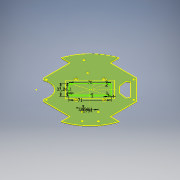
# Autodesk Inventor part: Board1.2
Saved by Autodesk Inventor 2020 (Build 240168000, 168)
## iProperties
Created: 2024-09-20
Part Number: Board1.2
Material: Типовые
Document SubType Name: Modeling
Designer: Ivan
Density: 1 g/cm^3
Appearance: Оливково-зеленый
Author: Ivan
Autodesk Inventor part; units mm, degrees
ref_plane "YZ Plane" through (0, 0, 0) normal (1, 0, 0) x (0, 1, 0)
ref_plane "XZ Plane" through (0, 0, 0) normal (0, 1, 0) x (-1, 0, 0)
ref_plane "XY Plane" through (0, 0, 0) normal (0, 0, 1) x (1, 0, 0)
sketch "Эскиз1" plane through (0, 0, 0) normal (0, 1, 0) x (-1, 0, 0)
  line L0 (-42.0023, -27.4404) -> (-27.4404, -42.0023)
  line L1 (-27.4404, -42.0023) -> (-25.1696, -59.5377)
  line L2 (-25.1696, -59.5377) -> (-32.6924, -63.2376)
  line L3 (-32.6924, -63.2376) -> (-63.2376, -32.6924)
  line L4 (-63.2376, -32.6924) -> (-59.5377, -25.1696)
  line L5 (-59.5377, -25.1696) -> (-42.0023, -27.4404)
  circle A0 centre (-72.43, 16) radius 3.3 construction
  circle A1 centre (44.87, -82.9015) radius 3.3 construction
  circle A2 centre (42.22, 16) radius 3.3
  circle A3 centre (-44.87, 82.9015) radius 3.3 construction
  circle A4 centre (-42.22, 16) radius 3.3 construction
  circle A5 centre (-82.9015, 44.87) radius 3.3 construction
  circle A6 centre (-16, 42.22) radius 3.3 construction
  circle A7 centre (72.43, -16) radius 3.3 construction
  circle A8 centre (16, -72.43) radius 3.3 construction
  circle A9 centre (-16, -72.43) radius 3.3 construction
  circle A10 centre (-42.22, -16) radius 3.3 construction
  circle A11 centre (16, -42.22) radius 3.3 construction
  circle A12 centre (16, 42.22) radius 3.3
  circle A13 centre (16, 72.43) radius 3.3 construction
  circle A14 centre (42.22, -16) radius 3.3 construction
  circle A15 centre (72.43, 16) radius 3.3 construction
  circle A16 centre (-16, 72.43) radius 3.3 construction
  circle A17 centre (82.9015, -44.87) radius 3.3 construction
  circle A18 centre (-16, -42.22) radius 3.3 construction
  circle A19 centre (-72.43, -16) radius 3.3 construction
  line L6 (31, 78.7724) -> (-31, 78.7724)
  line L7 (-31, 78.7724) -> (-31, 99.2724)
  arc A20 (-31, 99.2724) -> (-99.2724, 31) centre (0, 0) ccw
  line L8 (-99.2724, 31) -> (-78.7724, 31)
  line L9 (-78.7724, 31) -> (-78.7724, -31)
  line L10 (-78.7724, -31) -> (-99.2724, -31)
  arc A21 (-99.2724, -31) -> (-98.0863, -34.57) centre (0, 0) ccw
  arc A22 (-34.57, -98.0863) -> (-98.0863, -34.57) centre (-109.0212, -109.0212) ccw
  arc A23 (-34.57, -98.0863) -> (-31, -99.2724) centre (0, 0) ccw
  line L11 (-31, -99.2724) -> (-31, -78.7724)
  line L12 (-31, -78.7724) -> (31, -78.7724)
  line L13 (31, -78.7724) -> (31, -99.2724)
  arc A24 (31, -99.2724) -> (99.2724, -31) centre (0, 0) ccw
  line L14 (99.2724, -31) -> (78.7724, -31)
  line L15 (78.7724, -31) -> (78.7724, 31)
  line L16 (78.7724, 31) -> (99.2724, 31)
  arc A25 (99.2724, 31) -> (98.0863, 34.57) centre (0, 0) ccw
  arc A26 (34.57, 98.0863) -> (98.0863, 34.57) centre (109.0212, 109.0212) ccw
  arc A27 (34.57, 98.0863) -> (31, 99.2724) centre (0, 0) ccw
  line L17 (31, 99.2724) -> (31, 78.7724)
  circle A28 centre (31, 72.43) radius 1.5
  circle A29 centre (72.43, 31) radius 1.5
  circle A30 centre (0, 0) radius 20
  circle A31 centre (-72.43, -31) radius 1.5
  circle A32 centre (-31, -72.43) radius 1.5
  line L18 (-55.8614, 32.5269) -> (-79.196, 55.8614)
  line L19 (-79.196, 55.8614) -> (-55.8614, 79.196)
  line L20 (-55.8614, 79.196) -> (-32.5269, 55.8614)
  line L21 (-32.5269, 55.8614) -> (-55.8614, 32.5269)
  line L22 (48.3138, -22.4528) -> (80.4592, -54.5982)
  line L23 (80.4592, -54.5982) -> (54.5982, -80.4592)
  line L24 (54.5982, -80.4592) -> (22.4528, -48.3138)
  line L25 (22.4528, -48.3138) -> (48.3138, -22.4528)
  line L26 (31, 78.7724) -> (78.7724, 31)
  circle A33 centre (31, 72.43) radius 3.5 construction
  circle A34 centre (72.43, 31) radius 1.5 construction
  circle A35 centre (72.43, 31) radius 3.5 construction
  arc A36 (35.3732, 74.3992) -> (74.3992, 35.3732) centre (63.1933, 63.1933) ccw
  line L27 (-47.7297, -10.253) -> (10.253, 47.7297)
  line L28 (10.253, 47.7297) -> (47.7297, 10.253)
  line L29 (47.7297, 10.253) -> (-10.253, -47.7297)
  line L30 (-10.253, -47.7297) -> (-47.7297, -10.253)
  line L31 (-32.5269, 55.8614) -> (-55.8614, 32.5269) construction
  line L32 (-47.7297, -10.253) -> (47.7297, 10.253) construction
  line L33 (-78.7724, -31) -> (-31, -78.7724)
  dimension "d0" = 7
  dimension "d1" = 7
  dimension "d2" = 82
  dimension "d3" = 53
  constraints: 68 end point, 37 centre point, 18 point on circle, 4 coincident, 3 parallel, 2 point on line, 2 tangent, 1 midpoint, 1 perpendicular
  measures "d0" diameter of A33
  measures "d1" diameter of A35
  measures "d2" distance of L28.end L29.end
  measures "d3" distance of L27.end L28.end
extrude "Выдавливание1" add sketch "Эскиз1" along normal blind 1.6 contours A2 L28 | L28 A12 | L26 A36 L15 L14 A24 L13 L12 L33 L9 L8 A20 L7 L6 | L18 L19 L20 L21 | L22 L23 L24 L25 picked at (42.169, 17.1845) picked at (17.1503, 42.0834)
sketch "Эскиз2" plane through (0, 0, 0) normal (0, 1, 0) x (1, 0, 0)
  circle A0 centre (26.7696, -48.3187) radius 1.397
  circle A1 centre (47.6038, -27.4845) radius 1.397
  line L0 (47.6038, -27.4845) -> (26.7696, -48.3187) construction
  line L1 (22.4528, -48.3138) -> (24.6136, -50.4746) construction
  line L2 (26.7696, -48.3187) -> (24.6136, -50.4746) construction
  line L3 (-47.7297, -10.253) -> (10.253, 47.7297) projected
  line L4 (47.7297, 10.253) -> (-10.253, -47.7297) projected
  point P0 (-22.4528, 48.3138)
  point P1 (-79.196, 55.8614)
  point P2 (79.196, -55.8614)
  dimension "d6" = 3.0558
  dimension "d8" = 29.464
  dimension "d9" = 2.794
  constraints: 6 end point, 2 centre point, 1 collinear, 1 equal radius, 1 perpendicular
  measures "d6" distance from line of L0 L1.start
  measures "d8" distance of L0.start L0.end
  measures "d9" diameter of A0
sketch "Эскиз4" plane through (0, 1.6, 0) normal (0, 1, 0) x (1, 0, 0)
  arc A0 (75.5134, -56.8864) -> (75.5134, -52.6437) centre (73.3921, -54.7651) ccw
  line L0 (75.5134, -52.6437) -> (57.1286, -34.259)
  arc A1 (57.1286, -34.259) -> (52.886, -34.259) centre (55.0073, -36.3803) ccw
  line L1 (52.886, -34.259) -> (34.5012, -52.6437)
  arc A2 (34.5012, -52.6437) -> (34.5012, -56.8864) centre (36.6225, -54.7651) ccw
  line L2 (34.5012, -56.8864) -> (52.886, -75.2712)
  arc A3 (52.886, -75.2712) -> (57.1286, -75.2712) centre (55.0073, -73.1498) ccw
  line L3 (57.1286, -75.2712) -> (75.5134, -56.8864)
  circle A4 centre (62.7855, -48.7546) radius 0.5
  circle A5 centre (55.0073, -73.8569) radius 1.6
  circle A6 centre (74.0992, -54.7651) radius 1.6
  circle A7 centre (55.0073, -35.6732) radius 1.6
  circle A8 centre (61.0177, -39.9158) radius 0.5
  circle A9 centre (55.7144, -41.6836) radius 0.5
  circle A10 centre (57.4822, -43.4513) radius 0.5
  circle A11 centre (59.2499, -45.2191) radius 0.5
  circle A12 centre (61.0177, -46.9869) radius 0.5
  circle A13 centre (43.6936, -64.311) radius 0.5
  circle A14 centre (41.9258, -62.5432) radius 0.5
  circle A15 centre (62.7855, -41.6836) radius 0.5
  circle A16 centre (59.2499, -38.148) radius 0.5
  circle A17 centre (53.9466, -39.9158) radius 0.5
  circle A18 centre (35.9154, -54.7651) radius 1.6
  circle A19 centre (40.1581, -60.7755) radius 0.5
  circle A20 centre (38.3903, -59.0077) radius 0.5
  circle A21 centre (64.5532, -50.5224) radius 0.5
  circle A22 centre (66.321, -45.2191) radius 0.5
  circle A23 centre (64.5532, -43.4513) radius 0.5
  circle A24 centre (68.0888, -46.9869) radius 0.5
  circle A25 centre (69.8565, -48.7546) radius 0.5
  circle A26 centre (71.6243, -50.5224) radius 0.5
  line L4 (47.7297, 10.253) -> (-10.253, -47.7297) projected
  line L5 (18.7383, -18.7383) -> (73.5391, -73.5391) construction
  arc A27 (31, -99.2724) -> (99.2724, -31) centre (0, 0) ccw projected
  line L6 (-31, -78.7724) -> (31, -78.7724) projected
  line L7 (78.7724, -31) -> (31, -78.7724) construction
  point P0 (55.0073, -54.7651)
  point P1 (54.8862, -54.8862)
  constraints: 27 centre point, 12 end point, 9 point on circle, 2 midpoint, 1 point on line
extrude "Выдавливание4" cut sketch "Эскиз4" against normal through all contours A5 | A6 | A7 | A18
sketch "Эскиз5" plane through (0, 0, 0) normal (0, -1, 0) x (1, 0, 0)
  circle A0 centre (-37.2462, -31.2924) radius 1.6
  circle A1 centre (-67.8823, -53.033) radius 1.6
  arc A2 (99.2724, 31) -> (31, 99.2724) centre (0, 0) ccw
  constraints: 3 centre point, 2 point on circle
extrude "Выдавливание5" cut sketch "Эскиз5" against normal through all
sketch "Эскиз6" plane through (0, 1.6, 0) normal (0, 1, 0) x (1, 0, 0)
  circle A0 centre (49.1515, 117.5129) radius 1.65
  circle A1 centre (49.1515, 117.5129) radius 3.35
  circle A2 centre (3.9014, 156.8484) radius 1.65
  circle A3 centre (80, 152.9999) radius 1.65
  circle A4 centre (34.7499, 192.3354) radius 1.65
  circle A5 centre (41.9507, 154.9241) radius 41.494
  line L0 (45.9767, 118.5821) -> (51.7025, 119.6842)
  arc A6 (39.3031, 113.5146) -> (45.9767, 118.5821) centre (26.7374, 136.9912) ccw
  arc A7 (51.7025, 119.6842) -> (59.7803, 117.456) centre (62.7338, 143.9197) ccw
  arc A8 (78.4993, 155.995) -> (82.5887, 163.3089) centre (57.5919, 172.4852) ccw
  circle A9 centre (80, 152.9999) radius 3.35
  arc A10 (81.5355, 142.4824) -> (78.2048, 150.1715) centre (55.7405, 135.8747) ccw
  arc A11 (5.402, 153.8533) -> (1.3126, 146.5394) centre (26.3095, 137.3631) ccw
  circle A12 centre (3.9014, 156.8484) radius 3.35
  arc A13 (2.3659, 167.3659) -> (5.6965, 159.6768) centre (28.1609, 173.9736) ccw
  arc A14 (32.1989, 190.1641) -> (24.1211, 192.3923) centre (21.1675, 165.9286) ccw
  circle A15 centre (34.7499, 192.3354) radius 3.35
  arc A16 (44.5983, 196.3336) -> (37.9247, 191.2662) centre (57.1641, 172.8571) ccw
  line L1 (39.3031, 113.5146) -> (59.7803, 117.456) construction
  line L2 (-47.0226, -10.253) -> (10.253, 47.0226) construction
  line L3 (2.3659, 167.3659) -> (59.7803, 117.456) construction
  line L4 (24.121, 192.3922) -> (81.5355, 142.4824) construction
  line L5 (1.3126, 146.5394) -> (44.5983, 196.3336) construction
  line L6 (82.5887, 163.3089) -> (39.3031, 113.5146) construction
  circle A17 centre (41.9507, 154.9241) radius 38.0979 construction
  line L7 (45.9767, 118.5821) -> (46.9111, 113.7277) construction
  line L8 (78.2048, 150.1715) -> (78.4993, 155.995) construction
  line L9 (41.9507, 154.9241) -> (80, 152.9999) construction
  line L10 (41.9507, 154.9241) -> (34.7499, 192.3354) construction
  line L11 (41.9507, 154.9241) -> (3.9014, 156.8484) construction
  line L12 (5.6965, 159.6768) -> (5.402, 153.8533) construction
  line L13 (32.1989, 190.1641) -> (37.9247, 191.2662) construction
  line L14 (41.9507, 154.9241) -> (49.1515, 117.5129) construction
  circle A18 centre (-37.8224, 4.5736) radius 3.3
  circle A19 centre (-4.5736, 37.8224) radius 3.3
  circle A20 centre (4.5736, -37.8224) radius 3.3
  circle A21 centre (37.8224, -4.5736) radius 3.3
  circle A22 centre (16, -49.72) radius 3.3
  line L15 (-37.8224, 4.5736) -> (-4.5736, 37.8224) construction
  line L16 (4.5736, -37.8224) -> (37.8224, -4.5736) construction
  line L17 (-21.198, 21.198) -> (21.198, -21.198) construction
  line L18 (-4.5736, 37.8224) -> (37.8224, -4.5736) construction
  point P0 (-47.6168, 71.9305)
  point P1 (-60.3824, 55.6528)
  point P2 (-60.3824, 22.3934)
  point P3 (-47.6168, 6.1158)
  point P4 (2.7831, 6.1158)
  point P5 (15.5487, 22.3934)
  point P6 (15.2441, 55.8587)
  point P7 (2.9104, 71.5855)
  point P8 (0, 0)
  point P9 (-47.6168, 71.9305)
  point P10 (-60.3824, 55.6528)
  point P11 (-60.3824, 22.3934)
  point P12 (-47.6168, 6.1158)
  point P13 (2.7831, 6.1158)
  point P14 (15.5487, 22.3934)
  point P15 (15.2441, 55.8587)
  point P16 (2.9104, 71.5855)
  point P17 (0, 0)
  dimension "d45" = 82.9881
  dimension "d43" = 3.3
  dimension "d44" = 6.7
  dimension "d46" = 26.6279
  dimension "d47" = 20.4772
  dimension "d48" = 3.7148
  dimension "d49" = 33.1603
  dimension "d50" = 50.338
  dimension "d51" = 16.5802
  dimension "d52" = 25.169
  dimension "d53" = 10.4265
  dimension "d54" = 10.4265
  dimension "d55" = 10.4265
  dimension "d56" = 10.4265
  dimension "d57" = 10.4265
  dimension "d58" = 10.4265
  dimension "d59" = 59.957
  dimension "d60" = 47.021
  constraints: 38 end point, 28 point on circle, 22 centre point, 13 equal radius, 9 perpendicular, 6 coincident, 4 equal length, 4 parallel, 3 midpoint, 1 tangent, 12 other
  measures "d43" diameter of A0
  measures "d44" diameter of A1
  measures "d46" radius of A6
  measures "d47" horizontal distance of L1.end L1.start
  measures "d48" distance from line of L1 L0.start
  measures "d49" distance from line of L4 L3.start
  measures "d50" distance from line of L5 L6.start
  measures "d51" distance from line of L3 point (41.951, 154.924)
  measures "d52" distance from line of L5 point (41.951, 154.924)
  measures "d53" distance from line of L9 L6.start
  measures "d54" distance from line of L9 A10.start
  measures "d55" distance from line of L10 A14.end
  measures "d56" distance from line of L10 L5.end
  measures "d57" distance from line of L11 L3.start
  measures "d58" distance from line of L14 L1.end
  measures "d59" distance from line of L15 L16.end
  measures "d60" distance from line of L18 L15.start
extrude "Выдавливание6" cut sketch "Эскиз6" against normal blind 10 contours A18 | A19 | A20 | A21
sketch "Эскиз7" plane through (0, 1.6, 0) normal (0, 1, 0) x (1, 0, 0)
  line L0 (-38.2545, -11.9501) -> (-11.9501, -38.2545)
  line L1 (-11.9501, -38.2545) -> (38.2545, 11.9501)
  line L2 (38.2545, 11.9501) -> (11.9501, 38.2545)
  line L3 (11.9501, 38.2545) -> (-38.2545, -11.9501)
  line L4 (-38.2545, -11.9501) -> (38.2545, 11.9501) construction
  line L5 (-11.9501, -38.2545) -> (11.9501, 38.2545) construction
  line L6 (47.0226, 10.253) -> (-10.253, -47.0226) construction
  line L7 (-47.7297, -10.253) -> (10.253, 47.7297) projected
  line L8 (-10.253, -47.7297) -> (-47.7297, -10.253) projected
  line L9 (10.253, 47.7297) -> (47.7297, 10.253) projected
  line L10 (47.7297, 10.253) -> (-10.253, -47.7297) projected
  line L11 (-38.2545, -11.9501) -> (-11.9501, -38.2545)
  line L12 (-11.9501, -38.2545) -> (38.2545, 11.9501)
  line L13 (38.2545, 11.9501) -> (11.9501, 38.2545)
  line L14 (11.9501, 38.2545) -> (-38.2545, -11.9501)
  line L15 (-38.2545, -11.9501) -> (38.2545, 11.9501) construction
  line L16 (-11.9501, -38.2545) -> (11.9501, 38.2545) construction
  line L17 (47.0226, 10.253) -> (-10.253, -47.0226) construction
  line L18 (37.5474, 11.9501) -> (11.9501, 37.5474)
  line L19 (11.9501, 37.5474) -> (-37.5474, -11.9501)
  line L20 (-37.5474, -11.9501) -> (-11.9501, -37.5474)
  line L21 (-11.9501, -37.5474) -> (37.5474, 11.9501)
  line L22 (37.5474, 11.9501) -> (-37.5474, -11.9501) construction
  line L23 (32.5976, 11.243) -> (-11.243, -32.5976)
  line L24 (0, 0) -> (31.7322, -31.7322) construction
  circle A0 centre (32.5976, 11.243) radius 1.5
  line L25 (0, 0) -> (31.7322, 31.7322) construction
  line L26 (0, 0) -> (-9.9, 29) construction
  circle A1 centre (11.243, 32.5976) radius 1.5
  circle A2 centre (-11.243, -32.5976) radius 1.5
  circle A3 centre (-32.5976, -11.243) radius 1.5
  point P0 (0, 0)
  point P1 (0, 0)
  point P2 (10.6773, -10.6773)
  point P3 (-4.9797, 4.9797)
  point P4 (0, 0)
  dimension "d63" = 37.2
  dimension "d64" = 71
  dimension "d67" = 37.2
  dimension "d68" = 71
  dimension "d69" = 36.2
  dimension "d70" = 70
  dimension "d71" = 4
  dimension "d72" = 3
  dimension "d73" = 3
  dimension "d74" = 3
  dimension "d75" = 4
  constraints: 46 end point, 10 parallel, 9 midpoint, 5 coincident, 4 centre point, 4 perpendicular, 3 symmetric about line, 2 point on line, 4 other
  measures "d63" distance of L0.start L0.end
  measures "d64" distance from line of L0 L1.end
  measures "d67" distance of L11.start L11.end
  measures "d68" distance from line of L11 L12.end
  measures "d69" distance of L20.end L19.end
  measures "d70" distance of L19.end L18.end
  measures "d71" distance from line of L18 L23.start
  measures "d72" distance from line of L21 point (10.677, -10.677)
  measures "d73" diameter of A0
  measures "d74" distance from line of L19 A1.centre
  measures "d75" distance from line of L20 L23.end
extrude "Выдавливание8" add sketch "Эскиз7" against normal up to surface (1.6 mm away) contours L3 L2 L1 L0 | L7 L9 L10 L8 | L21 L20 L19 L18 | A0 | A1 | A2 | A3
hole "Отверстие1" at (-32.5976, 1.6, 11.243) at (11.243, 1.6, -32.5976) at (32.5976, 1.6, -11.243) at (-11.243, 1.6, 32.5976) direction (0, -1, 0) diameter 3 end through all
sketch "Эскиз8" plane through (0, 1.6, 0) normal (0, 1, 0) x (1, 0, 0)
  circle A0 centre (32.5976, 11.243) radius 1.5 projected
  circle A1 centre (-32.5976, -11.243) radius 1.5 projected
  circle A2 centre (11.243, 32.5976) radius 1.5 projected
  circle A3 centre (-11.243, -32.5976) radius 1.5 projected
  circle A4 centre (37.8224, -4.5736) radius 3.3 projected
  circle A5 centre (-4.5736, 37.8224) radius 3.3 projected
  circle A6 centre (4.5736, -37.8224) radius 3.3 projected
  circle A7 centre (-37.8224, 4.5736) radius 3.3 projected
  circle A8 centre (-37.2462, 31.2924) radius 1.6 projected
  circle A9 centre (-67.8823, 53.033) radius 1.6 projected
  circle A10 centre (55.0073, -73.8569) radius 1.6 projected
  circle A11 centre (74.0992, -54.7651) radius 1.6 projected
  circle A12 centre (35.9154, -54.7651) radius 1.6 projected
  circle A13 centre (55.0073, -35.6732) radius 1.6 projected
  arc A14 (-31, 99.2724) -> (-99.2724, 31) centre (0, 0) ccw projected
  line L0 (-99.2724, 31) -> (-78.7724, 31) projected
  line L1 (-78.7724, 31) -> (-78.7724, -31) projected
  line L2 (-78.7724, -31) -> (-74.3992, -35.3732) projected
  arc A15 (-35.3732, -74.3992) -> (-74.3992, -35.3732) centre (-63.1933, -63.1933) ccw projected
  line L3 (-35.3732, -74.3992) -> (-31, -78.7724) projected
  line L4 (-31, -78.7724) -> (31, -78.7724) projected
  line L5 (31, -78.7724) -> (31, -99.2724) projected
  arc A16 (31, -99.2724) -> (99.2724, -31) centre (0, 0) ccw projected
  line L6 (99.2724, -31) -> (78.7724, -31) projected
  line L7 (78.7724, -31) -> (78.7724, 31) projected
  line L8 (78.7724, 31) -> (31, 78.7724) projected
  line L9 (31, 78.7724) -> (-31, 78.7724) projected
  line L10 (-31, 78.7724) -> (-31, 99.2724) projected
  circle A17 centre (31, 72.43) radius 1.5 projected
  circle A18 centre (-72.43, -31) radius 1.5 projected
  line L11 (42.0023, 27.4404) -> (27.4404, 42.0023) projected
  line L12 (27.4404, 42.0023) -> (25.1696, 59.5377) projected
  line L13 (25.1696, 59.5377) -> (32.6924, 63.2376) projected
  line L14 (32.6924, 63.2376) -> (63.2376, 32.6924) projected
  line L15 (63.2376, 32.6924) -> (59.5377, 25.1696) projected
  line L16 (59.5377, 25.1696) -> (42.0023, 27.4404) projected
  circle A19 centre (-31, -72.43) radius 1.5 projected
  circle A20 centre (72.43, 31) radius 1.5 projected
equation "\"d53\" = d58"
equation "\"d54\" = d58"
equation "\"d55\" = d58"
equation "\"d56\" = d58"
equation "\"d57\" = d58"
